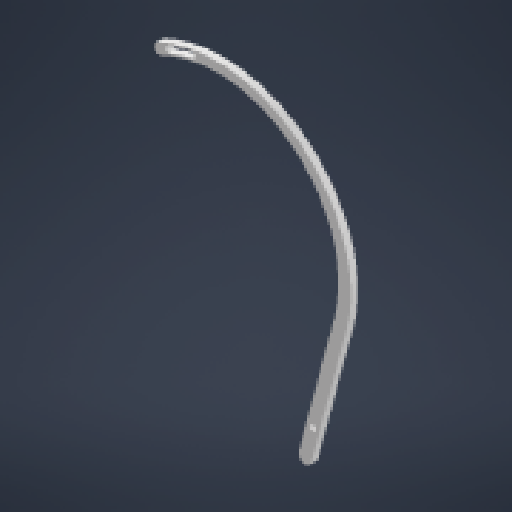
# Autodesk Inventor part: front rails
Saved by Autodesk Inventor 2025.2 (Build 292293000, 293)
## iProperties
Created: 2026-01-04
Part Number: front rails
Material: Acetal Resin, Black
Document SubType Name: Modeling
Designer: cloudy
Density: 1.425 g/cm^3
Appearance: Smooth - Black
Author: cloudy
Autodesk Inventor part; units mm, degrees
ref_plane "YZ Plane" through (0, 0, 0) normal (1, 0, 0) x (0, 1, 0)
ref_plane "XZ Plane" through (0, 0, 0) normal (0, 1, 0) x (-1, 0, 0)
ref_plane "XY Plane" through (0, 0, 0) normal (0, 0, 1) x (1, 0, 0)
sketch "Sketch1" plane through (0, 0, 0) normal (0, 0, 1) x (1, 0, 0)
  circle A0 centre (156.9617, 108.3117) radius 2.1844
  line L0 (171.7435, 196.3872) -> (150.4677, 101.0806)
  arc A1 (171.7435, 196.3872) -> (41.593, 297.4287) centre (78.8791, 211.1131) ccw
  arc A2 (152.3136, 109.3493) -> (161.5702, 107.1104) centre (156.9617, 108.3117) ccw
  line L1 (150.4677, 101.0806) -> (158.4911, 103.8014)
  line L2 (180.8293, 193.3835) -> (161.5702, 107.1104)
  circle A3 centre (40.3856, 300.9489) radius 2.1844 projected
  arc A4 (180.8293, 193.3835) -> (38.7207, 304.2652) centre (83.4742, 215.1165) ccw
  arc A5 (56.9002, 306.3451) -> (27.9409, 294.5249) centre (78.8791, 211.1131) ccw construction
  arc A6 (56.4089, 308.4736) -> (39.5252, 302.9567) centre (78.8791, 211.1131) ccw
  arc A7 (57.3914, 304.2167) -> (41.2459, 298.941) centre (78.8791, 211.1131) ccw
  arc A8 (57.3914, 304.2167) -> (56.4089, 308.4736) centre (56.9002, 306.3451) ccw
  arc A9 (39.5252, 302.9567) -> (41.2459, 298.941) centre (40.3856, 300.9489) ccw
  line L3 (83.4742, 215.1165) -> (56.9002, 306.3451) construction
  arc A10 (41.5411, 297.4113) -> (41.593, 297.4287) centre (40.3856, 300.9489) ccw
  line L4 (40.3856, 300.9489) -> (84.3253, 219.1399) construction
  arc A11 (38.7207, 304.2652) -> (42.1414, 297.6798) centre (40.3856, 300.9489) ccw
  line L5 (171.7435, 196.3872) -> (180.8293, 193.3835) construction
  point P0 (0, 0)
  point P1 (165.3829, 124.1896)
  point P2 (27.4473, 296.7796)
  point P3 (41.1972, 299.4378)
  point P4 (41.8471, 297.538)
  point P5 (41.2459, 298.941)
  point P6 (39.5252, 302.9567)
  dimension "d0" = 9.525
  dimension "d1" = 0
  dimension "d7" = 12
  constraints: 24 point on circle, 12 end point, 11 centre point, 9 tangent, 5 point on line, 4 coincident, 2 concentric, 1 parallel, 1 other
  measures "d0" diameter of A2
  measures "d1" distance of point (156.962, 108.312) A2.centre
  measures "d7" angle of L4 L3
extrude "Extrusion1" add sketch "Sketch1" along normal blind 7.62
body "Solid1"
